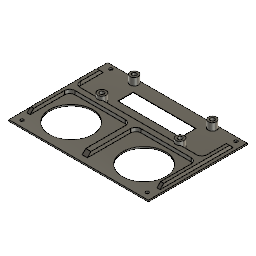
smmb_front-lcd-buttons (Autodesk Fusion 360 design; units mm, degrees)
Autodesk Fusion 360 part; units mm, degrees
sketch "Sketch1" plane through (0, 0, 0) normal (0, 0, 1) x (1, 0, 0)
  line L0 (0, 0) -> (134, 0)
  line L1 (134, 0) -> (134, 95)
  line L2 (134, 95) -> (0, 95)
  line L3 (0, 95) -> (0, 0)
  line L4 (27, 93.45) -> (107, 93.45)
  line L5 (107, 93.45) -> (107, 57.45)
  line L6 (107, 57.45) -> (27, 57.45)
  line L7 (27, 57.45) -> (27, 93.45)
  line L8 (37, 82.45) -> (97, 82.45)
  line L9 (97, 82.45) -> (97, 67.95)
  line L10 (97, 67.95) -> (37, 67.95)
  line L11 (37, 67.95) -> (37, 82.45)
  circle A0 centre (7, 91) radius 1.55
  circle A1 centre (127, 91) radius 1.55
  circle A2 centre (127, 6) radius 1.55
  circle A3 centre (7, 6) radius 1.55
  line L12 (29.5, 90.95) -> (104.5, 90.95)
  line L13 (104.5, 90.95) -> (104.5, 59.95)
  line L14 (104.5, 59.95) -> (29.5, 59.95)
  line L15 (29.5, 59.95) -> (29.5, 90.95)
  circle A4 centre (29.5, 90.95) radius 2.05
  circle A5 centre (29.5, 90.95) radius 4.05
  circle A6 centre (104.5, 90.95) radius 2.05
  circle A7 centre (104.5, 90.95) radius 4.05
  circle A8 centre (104.5, 59.95) radius 2.05
  circle A9 centre (104.5, 59.95) radius 4.05
  circle A10 centre (29.5, 59.95) radius 2.05
  circle A11 centre (29.5, 59.95) radius 4.05
  circle A12 centre (102, 28) radius 22.5
  circle A13 centre (102, 28) radius 12.25
  circle A14 centre (32, 28) radius 9
  circle A15 centre (32, 28) radius 8.25
  line L16 (0, 47) -> (0, 52.45)
  line L17 (3.2, 52) -> (3.2, 47)
  line L18 (130.8, 52) -> (130.8, 47)
  line L19 (6.2, 84.5) -> (3.2, 84.5)
  line L20 (3.2, 84.5) -> (3.2, 14.5)
  line L21 (3.2, 14.5) -> (6.2, 14.5)
  line L22 (6.2, 14.5) -> (6.2, 84.5)
  line L23 (6.2, 84.5) -> (3.2, 14.5) construction
  line L24 (3.2, 84.5) -> (6.2, 14.5) construction
  line L25 (130.8, 14.5) -> (127.8, 14.5)
  line L26 (127.8, 14.5) -> (127.8, 84.5)
  line L27 (127.8, 84.5) -> (130.8, 84.5)
  line L28 (130.8, 84.5) -> (130.8, 14.5)
  line L29 (130.8, 14.5) -> (127.8, 84.5) construction
  line L30 (127.8, 14.5) -> (130.8, 84.5) construction
  circle A16 centre (102, 28) radius 9
  circle A17 centre (102, 28) radius 8.25
  circle A18 centre (32, 28) radius 12.25
  circle A19 centre (32, 28) radius 22.5
  line L31 (67, 57.45) -> (67, 0)
  circle A20 centre (32, 28) radius 20.625
  circle A21 centre (102, 28) radius 20.625
  line L32 (69.5, 0) -> (64.5, 0)
  line L33 (64.5, 0) -> (64.5, 57.45)
  line L34 (64.5, 57.45) -> (69.5, 57.45)
  line L35 (69.5, 57.45) -> (69.5, 0)
  line L36 (69.5, 0) -> (64.5, 57.45) construction
  line L37 (64.5, 0) -> (69.5, 57.45) construction
  line L38 (0, 57.45) -> (134, 57.45)
  line L39 (134, 57.45) -> (134, 52.45)
  line L40 (134, 52.45) -> (0, 52.45)
  line L41 (0, 52.45) -> (0, 57.45)
  line L42 (0, 57.45) -> (134, 52.45) construction
  line L43 (134, 57.45) -> (0, 52.45) construction
  line L44 (127, 6) -> (7, 6)
  point P0 (4.7, 49.5)
  point P1 (129.3, 49.5)
  point P2 (67, 28.725)
  point P3 (67, 54.95)
  dimension "d1" = 134
  dimension "d2" = 95
  dimension "d3" = 80
  dimension "d4" = 36
  dimension "d5" = 27
  dimension "d6" = 1.55
  dimension "d7" = 60
  dimension "d8" = 14.5
  dimension "d9" = 11
  dimension "d10" = 10
  dimension "d11" = 3.1
  dimension "d12" = 7
  dimension "d13" = 4
  dimension "d14" = 3.1
  dimension "d15" = 7
  dimension "d16" = 4
  dimension "d17" = 3.1
  dimension "d18" = 7
  dimension "d19" = 6
  dimension "d20" = 3.1
  dimension "d21" = 7
  dimension "d22" = 6
  dimension "d23" = 75
  dimension "d24" = 31
  dimension "d25" = 2.5
  dimension "d26" = 2.5
  dimension "d27" = 4.1
  dimension "d28" = 8.1
  dimension "d29" = 4.1
  dimension "d30" = 4.1
  dimension "d31" = 4.1
  dimension "d32" = 8.1
  dimension "d33" = 8.1
  dimension "d34" = 8.1
  dimension "d35" = 45
  dimension "d36" = 24.5
  dimension "d37" = 18
  dimension "d38" = 16.5
  dimension "d39" = 70
  dimension "d40" = 32
  dimension "d42" = 28
  dimension "d43" = 28
  dimension "d46" = 3.2
  dimension "d47" = 3.2
  dimension "d50" = 3
  dimension "d51" = 70
  dimension "d52" = 70
  dimension "d53" = 3
  dimension "d60" = 18
  dimension "d61" = 16.5
  dimension "d62" = 24.5
  dimension "d63" = 45
  dimension "d70" = 41.25
  dimension "d71" = 41.25
  dimension "d72" = 4.7
  dimension "d73" = 4.7
  dimension "d75" = 5
  dimension "d76" = 5
  dimension "d77" = 2.5
  constraint horizontal L0
  constraint vertical L1
  constraint horizontal L2
  constraint vertical L3
  constraint coincident L0.start L3.end
  constraint horizontal L4
  constraint vertical L5
  constraint horizontal L6
  constraint vertical L7
  constraint horizontal L8
  constraint vertical L9
  constraint horizontal L10
  constraint vertical L11
  constraint horizontal L12
  constraint vertical L13
  constraint horizontal L14
  constraint vertical L15
  constraint coincident L12.start L15.end
  constraint concentric A4 A5
  constraint coincident L12.end L13.start
  constraint concentric A6 A7
  constraint coincident L13.end L14.start
  constraint concentric A8 A9
  constraint coincident L14.end L15.start
  constraint concentric A10 A11
  constraint concentric A12 A13
  constraint concentric A14 A15
  constraint vertical L16
  constraint coincident L3 L16.end
  constraint perpendicular L19 L20
  constraint parallel L19 L21
  constraint parallel L20 L22
  constraint horizontal L19
  constraint coincident L23 P0
  constraint coincident L24 P0
  constraint perpendicular L25 L26
  constraint parallel L25 L27
  constraint parallel L26 L28
  constraint horizontal L25
  constraint coincident L29 P1
  constraint coincident L30 P1
  constraint concentric A13 A16
  constraint concentric A12 A17
  constraint concentric A14 A18
  constraint concentric A14 A19
  constraint midpoint L0 L31.end
  constraint perpendicular L0 L31
  constraint concentric A15 A20
  constraint concentric A13 A21
  constraint coincident L6 L31.start
  constraint perpendicular L32 L33
  constraint parallel L32 L34
  constraint parallel L33 L35
  constraint horizontal L32
  constraint coincident L0 L32.start
  constraint coincident L36 P2
  constraint coincident L37 P2
  constraint midpoint L31 P2
  constraint perpendicular L38 L39
  constraint parallel L38 L40
  constraint parallel L39 L41
  constraint horizontal L38
  constraint coincident L3 L38.start
  constraint coincident L42 P3
  constraint coincident L43 P3
  constraint coincident L31 P3
  constraint coincident A2.centre L44.start
  constraint coincident A3.centre L44.end
  measures "d1" distance of L0.start L0.end
  measures "d2" distance of L0.start L2.end
  measures "d3" distance of L4.start L4.end
  measures "d4" distance of L4.start L6.end
  measures "d5" distance of L3 L7
  measures "d6" distance of L2 L4
  measures "d7" distance of L8.start L8.end
  measures "d8" distance of L8.start L10.end
  measures "d9" distance of L4 L8
  measures "d10" distance of L7 L11
  measures "d11" diameter of A0
  measures "d12" distance of L3 A0.centre
  measures "d13" distance of L2 A0.centre
  measures "d14" diameter of A1
  measures "d15" distance of L1 A1.centre
  measures "d16" distance of L2 A1.centre
  measures "d17" diameter of A2
  measures "d18" distance of L1 A2.centre
  measures "d19" distance of L0 A2.centre
  measures "d20" diameter of A3
  measures "d21" distance of L3 A3.centre
  measures "d22" distance of L0 A3.centre
  measures "d23" distance of L12.start L12.end
  measures "d24" distance of L12.start L14.end
  measures "d25" distance of L7 L15
  measures "d26" distance of L4 L12
  measures "d27" diameter of A4
  measures "d28" diameter of A5
  measures "d29" diameter of A10
  measures "d30" diameter of A6
  measures "d31" diameter of A8
  measures "d32" diameter of A11
  measures "d33" diameter of A7
  measures "d34" diameter of A9
  measures "d35" diameter of A12
  measures "d36" diameter of A13
  measures "d37" diameter of A14
  measures "d38" diameter of A15
  measures "d39" distance of A12.centre A14.centre
  measures "d40" distance of L3 A14.centre
  measures "d42" distance of L0 A12.centre
  measures "d43" distance of L0 A14.centre
  measures "d46" distance of L16 L17
  measures "d47" distance of L1 L18
  measures "d50" distance of L20.end L21.end
  measures "d51" distance of L19.end L20.end
  measures "d52" distance of L25.end L26.end
  measures "d53" distance of L26.end L27.end
  measures "d60" diameter of A16
  measures "d61" diameter of A17
  measures "d62" diameter of A18
  measures "d63" diameter of A19
  measures "d70" diameter of A20
  measures "d71" diameter of A21
  measures "d72" distance of L3 P0
  measures "d73" distance of L1 P1
  measures "d75" distance of L33.end L34.end
  measures "d76" distance of L38.end L39.end
  measures "d77" distance of L31.start P3
extrude "Extrude1" add sketch "Sketch1" along normal blind 1.5 contours L0 L3 L16 L17 L20 L21 L22 L33 L40 | L0 L31 L32 L33 L44 | L0 L31 L32 L35 L44 | L31 L33 L40 L44 | L3 L20 L38 L40 L41 | L0 L1 L18 L25 L26 L28 L35 L40 | L31 L35 L40 L44 | L6 A11 L22 L33 L38 L40 | L6 L31 L33 L34 L38 L40 | L2 L3 L7 A5 A11 L19 L20 L22 L38 | L17 L20 L21 L22 L40 | L20 L22 L38 L40 | L6 L31 L34 L35 L38 L40 | L6 L14 A9 A11 L34 L38 | L19 L20 L22 L38 | L1 L28 L38 L39 L40 | L6 A9 L26 L35 L38 L40 | L6 A11 L38 | L6 L7 L14 L15 A10 A11 L38 | L2 L4 A5 A7 | L4 L7 A5 | L1 L2 L5 A7 A9 L26 L27 L28 L38 | L26 L28 L38 L40 | L18 L25 L26 L28 L40 | L7 A11 L38 | L12 L13 L14 L15 A5 A7 A9 A11 | L14 L15 A10 A11 | L4 L5 A7 | L4 L7 L12 L15 A4 A5 | L4 L12 A5 A7 | L7 L15 A5 A11 | L26 L27 L28 L38 | L5 L6 L13 L14 A8 A9 L38 | L6 A9 L38 | L14 L15 A10 | L14 L15 A10 | L13 L14 A8 A9 | L4 L5 L12 L13 A6 A7 | L12 L15 A4 A5 | L5 A9 L38 | L13 L14 A8 | L13 L14 A8 | L5 L13 A7 A9 | L12 L13 A6 A7 | L12 L15 A4 | L12 L15 A4 | L12 L13 A6 | L12 L13 A6 | A12 L44 | A12 L44 | A19 L44 | A19 L44
extrude "Extrude2" add sketch "Sketch1" along normal blind 5 contours L31 L33 L40 L44 | L31 L35 L40 L44 | L6 A11 L22 L33 L38 L40 | L6 L31 L33 L34 L38 L40 | L17 L20 L21 L22 L40 | L20 L22 L38 L40 | L6 L31 L34 L35 L38 L40 | L19 L20 L22 L38 | L6 A9 L26 L35 L38 L40 | L26 L28 L38 L40 | L18 L25 L26 L28 L40 | L26 L27 L28 L38
extrude "Extrude3" add sketch "Sketch1" along normal blind 8.5 contours L6 A11 L38 | L6 L7 L14 L15 A10 A11 L38 | L4 L7 A5 | L7 A11 L38 | L14 L15 A10 A11 | L4 L5 A7 | L4 L7 L12 L15 A4 A5 | L5 L6 L13 L14 A8 A9 L38 | L6 A9 L38 | L13 L14 A8 A9 | L4 L5 L12 L13 A6 A7 | L12 L15 A4 A5 | L5 A9 L38 | L12 L13 A6 A7
chamfer "Chamfer1" distance 1 angle 45 4 edges at (67, 82.45, 0) (97, 75.2, 0) (67, 67.95, 0) (37, 75.2, 0)
fillet "Fillet2" radius 5 6 edges at (6.2, 52.45, 3.25) (6.2, 57.45, 3.25) (64.5, 52.45, 3.25) (69.5, 52.45, 3.25) (127.8, 52.45, 3.25) (127.8, 57.45, 3.25)
chamfer "Chamfer4" distance 3.5 angle 45 5 edges at (4.7, 84.5, 5) (4.7, 14.5, 5) (67, 6, 5) (129.3, 14.5, 5) (129.3, 84.5, 5)
equation "d5 = d1 / 2 - d3 / 2"
equation "d6 = 4 mm - 2.45 mm"
equation "d10 = d3 / 2 - d7 / 2"
equation "d14 = d11"
equation "d17 = d11"
equation "d20 = d11"
equation "d26 = d25"
equation "d28 = d27 + 4 mm"
equation "d29 = d27"
equation "d30 = d27"
equation "d31 = d27"
equation "d32 = d28"
equation "d33 = d28"
equation "d34 = d28"
equation "d43 = d42"
equation "d58 = 1.5 mm + 7 mm"
